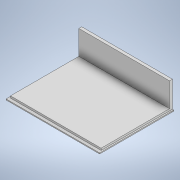
# Autodesk Inventor part: Крышка Корпуса3
Saved by Autodesk Inventor 2021.2 (Build 252289000, 289)
## iProperties
Created: 2023-02-07
Part Number: Крышка Корпуса3
Material: Типовые
Document SubType Name: Modeling
Designer: Wyvern
Density: 1 g/cm^3
Appearance: По умолчанию
Author: Wyvern
Autodesk Inventor part; units mm, degrees
ref_plane "YZ Plane" through (0, 0, 0) normal (1, 0, 0) x (0, 1, 0)
ref_plane "XZ Plane" through (0, 0, 0) normal (0, 1, 0) x (-1, 0, 0)
ref_plane "XY Plane" through (0, 0, 0) normal (0, 0, 1) x (1, 0, 0)
sketch "Эскиз1" plane through (0, 0, 0) normal (0, 1, 0) x (-1, 0, 0)
  line L0 (-48.5, 38.5) -> (48.5, 38.5)
  line L1 (48.5, 38.5) -> (48.5, -38.5)
  line L2 (48.5, -38.5) -> (-48.5, -38.5)
  line L3 (-48.5, -38.5) -> (-48.5, 38.5)
  line L4 (-48.5, 38.5) -> (48.5, -38.5) construction
  line L5 (48.5, 38.5) -> (-48.5, -38.5) construction
  point P0 (0, 0)
  dimension "d0" = 77
  dimension "d1" = 97
  constraints: 12 end point, 2 midpoint, 2 parallel, 1 horizontal, 1 perpendicular
  measures "d0" distance of L0.end L1.end
  measures "d1" distance of L0.start L0.end
extrude "Выдавливание1" add sketch "Эскиз1" along normal blind 1
sketch "Эскиз2" plane through (0, 1, 0) normal (0, 1, 0) x (1, 0, 0)
  line L0 (48.5, 38.5) -> (-48.5, 38.5) projected
  line L1 (-47, 38.5) -> (47, 38.5)
  line L2 (47, 38.5) -> (47, -35.5)
  line L3 (47, -35.5) -> (-47, -35.5)
  line L4 (-47, -35.5) -> (-47, 38.5)
  line L5 (0, 38.5) -> (0, 0)
  line L6 (-48.5, -38.5) -> (48.5, -38.5) projected
  dimension "d4" = 94
  dimension "d5" = 3
  constraints: 10 end point, 2 parallel, 1 horizontal, 1 midpoint, 1 perpendicular, 1 point on line, 1 vertical, 1 other
  measures "d4" distance between parallel lines of L4 L2
  measures "d5" distance between parallel lines of L6 L3
extrude "Выдавливание2" add sketch "Эскиз2" along normal blind 2
sketch "Эскиз3" plane through (0, 3, 0) normal (0, 1, 0) x (1, 0, 0)
  line L0 (47, 38.5) -> (-47, 38.5) projected
  line L1 (47, 38.5) -> (47, -35.5) projected
  line L2 (-47, 38.5) -> (47, 38.5)
  line L3 (47, 38.5) -> (47, 35.5)
  line L4 (47, 35.5) -> (-47, 35.5)
  line L5 (-47, 35.5) -> (-47, 38.5)
  point P0 (0, 0)
  dimension "d8" = 3
  constraints: 8 end point, 2 parallel, 1 horizontal, 1 perpendicular, 1 point on line
  measures "d8" distance between parallel lines of L0 L4
extrude "Выдавливание3" add sketch "Эскиз3" along normal blind 25
